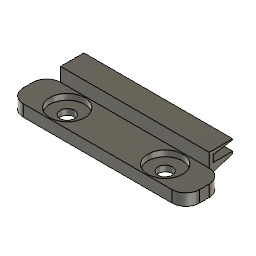
toteRack (Autodesk Fusion 360 design; units mm, degrees)
part number: 2026-08-10-19-56-16-923
Autodesk Fusion 360 part; units mm, degrees
sketch "Sketch1" plane through (0, 0, 0) normal (0, 0, 1) x (1, 0, 0)
  line L0 (-28, 37) -> (62, 37)
  line L1 (62, 37) -> (62, 18)
  line L2 (62, 18) -> (-28, 18)
  line L3 (-28, 18) -> (-28, 37)
  dimension "d1" = 90
  dimension "d2" = 19
  constraint horizontal L0
  constraint vertical L1
  constraint horizontal L2
  constraint vertical L3
  measures "d1" distance of L0.start L0.end
  measures "d2" distance of L0.start L2.end
extrude "Extrude1" add sketch "Sketch1" along normal blind 6
fillet "Fillet1" radius 7 3 edges at (62, 37, 3) (62, 18, 3) (-28, 18, 3)
fillet "Fillet2" radius 7 1 edges at (-28, 37, 3)
sketch "Sketch2" plane through (0, 0, 6) normal (0, 0, 1) x (-1, 0, 0)
  arc A0 (21, -37) -> (28, -30) centre (21, -30) ccw
  line L0 (28, -30) -> (28, -25)
  arc A1 (28, -25) -> (21, -18) centre (21, -25) ccw
  line L1 (21, -18) -> (-55, -18)
  arc A2 (-55, -18) -> (-62, -25) centre (-55, -25) ccw
  line L2 (-62, -25) -> (-62, -30)
  arc A3 (-62, -30) -> (-55, -37) centre (-55, -30) ccw
  line L3 (-55, -37) -> (21, -37)
ref_plane "WorkPlane1" through (17, 27.5, 6) normal (0, 0, 1) x (-1, 0, 0)
sketch "Sketch3" plane through (0, 0, 6) normal (0, 0, 1) x (1, 0, 0)
  line L0 (17, 37) -> (17, 18)
  circle A0 centre (-8, 27.5) radius 8.9
  circle A1 centre (42, 27.5) radius 8.9
  circle A2 centre (-8, 27.5) radius 3.65
  circle A3 centre (42, 27.5) radius 3.65
  dimension "d13" = 17.8
  dimension "d14" = 17.8
  dimension "d15" = 7.3
  dimension "d16" = 7.3
  constraint vertical L0
  constraint concentric A0 A2
  constraint concentric A1 A3
  measures "d13" diameter of A0
  measures "d14" diameter of A1
  measures "d15" diameter of A2
  measures "d16" diameter of A3
extrude "Extrude2" cut sketch "Sketch3" against normal blind 7 contours A2 | A3
extrude "Extrude3" cut sketch "Sketch3" against normal blind 3
sketch "Sketch4" plane through (0, 0, 0) normal (0, 0, 1) x (1, 0, 0)
  line L0 (-21, 37) -> (55, 37)
  line L1 (55, 37) -> (55, 39)
  line L2 (55, 39) -> (-21, 39)
  line L3 (-21, 39) -> (-21, 37)
  dimension "d21" = 76
  dimension "d22" = 2
  constraint horizontal L0
  constraint vertical L1
  constraint horizontal L2
  constraint vertical L3
  measures "d21" distance of L0.start L0.end
  measures "d22" distance of L0.start L2.end
extrude "Extrude4" add sketch "Sketch4" along normal blind 13
ref_plane "WorkPlane2" through (-21, 38, 6.5) normal (-1, 0, 0) x (0, -1, 0)
sketch "Sketch5" plane through (-21, 0, 0) normal (-1, 0, 0) x (0, -1, 0)
  line L0 (-39, 13) -> (-49, 13)
  line L1 (-49, 13) -> (-49, 12)
  line L2 (-39, 13) -> (-39, 11)
  line L3 (-49, 12.5) -> (-39, 11)
  dimension "d26" = 10
  dimension "d27" = 1
  constraint horizontal L0
  constraint perpendicular L0 L1
  constraint perpendicular L0 L2
  constraint midpoint L1 L3.start
  measures "d26" distance of L0.start L0.end
  measures "d27" distance of L0.end L1.end
extrude "Extrude5" add sketch "Sketch5" against normal blind 76
sketch "Sketch6" plane through (-21, 0, 0) normal (-1, 0, 0) x (0, -1, 0)
  line L0 (-39, 0) -> (-37, 0)
  line L1 (-37, 0) -> (-37, 6)
  line L2 (-37, 6) -> (-37, 13)
  line L3 (-37, 13) -> (-49, 13)
  line L4 (-49, 13) -> (-49, 12.5)
  line L5 (-49, 12.5) -> (-39, 11)
  line L6 (-39, 11) -> (-39, 0)
  line L7 (-39, 7.5) -> (-49, 7.5)
  line L8 (-49, 7.5) -> (-49, 6.3428)
  line L9 (-49, 6.3428) -> (-39, 3.3342)
  line L10 (-39, 7.5) -> (-39, 3.3342)
  dimension "d34" = 10
  constraint coincident L6 L7.start
  constraint perpendicular L6 L7
  constraint perpendicular L7 L8
  constraint coincident L6 L9.end
  measures "d34" distance of L7.start L7.end
extrude "Extrude6" add sketch "Sketch6" against normal blind 76 contours L6 L7 L8 L9 L10
